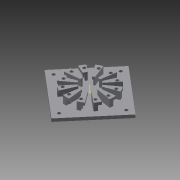
# Autodesk Inventor part: male bayonet connector 12
Saved by Autodesk Inventor 2015 (Build 190159000, 159)
## iProperties
Created: 2014-06-11
Part Number: male bayonet connector 12
Material: Generic
Document SubType Name: Modeling
Designer: ericd_000
Density: 1 g/cm^3
Appearance: Default
Author: ericd_000
Autodesk Inventor part; units mm, degrees
ref_plane "YZ Plane" through (0, 0, 0) normal (1, 0, 0) x (0, 1, 0)
ref_plane "XZ Plane" through (0, 0, 0) normal (0, 1, 0) x (-1, 0, 0)
ref_plane "XY Plane" through (0, 0, 0) normal (0, 0, 1) x (1, 0, 0)
sketch "Sketch19" plane through (0, 0, 0) normal (0, 0, 1) x (1, 0, 0)
  circle A0 centre (0, 0) radius 39.5
  dimension "d94" = 79
  constraints: 1 centre point, 1 coincident
  measures "d94" diameter of A0
extrude "Extrusion20" add sketch "Sketch19" along normal blind 5
sketch "Sketch21" plane through (0, 0, 5) normal (0, 0, 1) x (1, 0, 0)
  point P0 (0, 0)
sketch "Sketch23" plane through (0, 0, 5) normal (0, 0, 1) x (1, 0, 0)
  line L0 (0, 0) -> (20.2843, 33.8939) construction
  circle A0 centre (0, 0) radius 39.5 construction
  line L1 (0, 0) -> (24.804, 30.7411) construction
  circle A1 centre (0, 0) radius 39.5 construction
  line L2 (24.804, 30.7411) -> (9.4735, 11.7411)
  line L3 (9.4735, 11.7411) -> (7.6719, 12.8193)
  line L4 (7.6719, 12.8193) -> (20.2843, 33.8939)
  arc A2 (24.804, 30.7411) -> (20.2843, 33.8939) centre (0, 0) ccw
  dimension "d105" = 172
  dimension "d106" = 19
  constraints: 10 end point, 2 collinear, 2 point on circle, 1 centre point, 1 perpendicular, 5 other
  measures "d105" angle of L0 L1
  measures "d106" vertical distance of L1.end L2.end
extrude "Extrusion21" add sketch "Sketch23" along normal blind 12.5
sketch "Sketch26" plane through (7.6719, 12.8193, 5) normal (-0.8580744, 0.5135254, 0) x (0, 0, 1)
  line L0 (12.5, 24.5604) -> (12.5, 0)
  line L1 (12.5, 24.5604) -> (8.1, 24.5604)
  line L2 (0, 24.5604) -> (12.5, 24.5604) projected
  line L3 (0, 0) -> (12.5, 0) projected
  line L4 (8.1, 0) -> (12.5, 0)
  line L5 (8.1, 24.5604) -> (8.1, 0)
  line L6 (-8.5, -14.9396) -> (16, -14.9396) projected
  line L7 (12.5, 24.5604) -> (12.5, 0) projected
  point P0 (-5, -14.9396)
  dimension "d123" = 4.4
  constraints: 8 end point, 2 point on line, 1 collinear, 1 parallel, 1 vertical
  measures "d123" distance of L4.start L0.end
revolve "Revolution2" add sketch "Sketch26" angle 7 about axis through (0, 0, 5) along (0, 0, 1)
sketch "Sketch25" plane through (0, 0, 17.5) normal (0, 0, 1) x (1, 0, 0)
  circle A0 centre (18.2106, 27.5205) radius 2.5
  line L0 (18.2106, 27.5205) -> (0, 0) construction
  line L1 (6.0524, 13.6587) -> (16.0024, 36.1133) projected
  dimension "d112" = 5
  dimension "d116" = 33
  dimension "d125" = 5.5
  constraints: 2 end point, 1 centre point
  measures "d112" diameter of A0
  measures "d116" distance of L0.start L0.end
  measures "d125" distance from line of L0.start L1
extrude "Extrusion22" cut sketch "Sketch25" against normal through all
sketch "Sketch27" plane through (0, 0, 17.5) normal (0, 0, 1) x (1, 0, 0)
  line L0 (7.6719, 12.8193) -> (9.4735, 11.7411) projected
  line L1 (7.6719, 12.8193) -> (6.0524, 13.6587)
  line L2 (6.0524, 13.6587) -> (20.1635, 45.5037)
  line L3 (6.0524, 13.6587) -> (16.0024, 36.1133) projected
  line L4 (20.1635, 45.5037) -> (7.6753, 12.8175)
  point P0 (0, 0)
  constraints: 7 end point, 2 point on line
extrude "Extrusion23" [suppressed]
pattern_circular "Circular Pattern2" count 12 over 360 about axis through (0, 0, 5) along (0, 0, 1) of "Extrusion21", "Revolution2", "Extrusion22"
sketch "Sketch29" plane through (0, 0, 5) normal (0, 0, 1) x (1, 0, 0)
  circle A0 centre (0, 0) radius 59
  line L0 (0, 0) -> (-30.7411, 24.804)
  line L1 (0, 0) -> (-33.8939, 20.2843)
  line L2 (-12.8193, 7.6719) -> (-33.8939, 20.2843) projected
  arc A1 (-34.5136, -19.2109) -> (-24.804, -30.7411) centre (0, 0) ccw projected
  point P0 (-30.0077, 17.9585)
  dimension "d135" = 118
  constraints: 4 end point, 1 centre point, 1 coincident, 1 collinear, 1 concentric
  measures "d135" diameter of A0
extrude "Extrusion26" [suppressed]
sketch "Sketch30" plane through (0, 0, 5) normal (0, 0, -1) x (-1, 0, 0)
  line L0 (-109.7485, 105.489) -> (97.8298, 105.489)
  line L1 (97.8298, 105.489) -> (97.8298, -69.3705)
  line L2 (97.8298, -69.3705) -> (-109.7485, -69.3705)
  line L3 (-109.7485, -69.3705) -> (-109.7485, 105.489)
  line L4 (10.1144, -4.0386) -> (9.0138, 1.6159)
  line L5 (9.0138, 1.6159) -> (50.6067, 20.2684)
  line L6 (50.6067, 20.2684) -> (50.6067, -5.7642)
  line L7 (50.6067, -5.7642) -> (10.1144, -4.0386)
  point P0 (0, 0)
  constraints: 16 end point, 2 parallel, 1 horizontal, 1 perpendicular, 1 vertical
extrude "Extrusion27" [suppressed]
sketch "Sketch31" plane through (-36.1133, 16.0024, 17.5) normal (0, 0, 1) x (0.9142614, -0.4051247, 0)
  line L0 (16, 0) -> (20, 0)
  line L1 (20, 0) -> (20, 3)
  line L2 (20, 3) -> (16, 3)
  line L3 (16, 3) -> (16, 0)
  line L4 (24.5604, 0) -> (0, 0) projected
  point P0 (39.5, 0)
  point P1 (24.7502, 0)
  dimension "d148" = 16
  dimension "d149" = 4
  dimension "d150" = 3
  constraints: 8 end point, 2 parallel, 1 collinear, 1 horizontal, 1 perpendicular
  measures "d148" distance from line of L3 L4.end
  measures "d149" distance of L1.end L2.end
  measures "d150" distance of L0.end L1.end
extrude "Extrusion28" cut sketch "Sketch31" against normal up to surface (4.4 mm away)
sketch "Sketch32" plane through (-30.7411, 24.804, 17.5) normal (0, 0, 1) x (0.7782548, -0.6279487, 0)
  line L0 (16.8007, -6.0822) -> (15.171, 0)
  line L1 (0, 0) -> (24.4136, 0) projected
  line L2 (16.8007, -6.0822) -> (16.0243, -3.1845) projected
  line L3 (16.8007, -6.0822) -> (25.0695, -3.8666)
  line L4 (25.0695, -3.8666) -> (24.4136, 0)
  line L5 (15.171, 0) -> (24.4136, 0)
  line L6 (16.8007, -6.0822) -> (16.511, -6.1599)
  line L7 (16.8007, -6.0822) -> (1.3459, -10.2234) projected
  line L8 (14.8604, 0) -> (15.171, 0)
  line L9 (15.171, 0) -> (14.8604, 0)
  line L10 (16.511, -6.1599) -> (14.8604, 0)
  point P0 (39.5, 0)
  point P1 (8.718, -8.248)
  dimension "d153" = 0.3
  constraints: 16 end point, 4 collinear, 3 point on line, 1 parallel
  measures "d153" distance between parallel lines of L10 L0
extrude "Extrusion30" cut sketch "Sketch32" against normal up to surface (12.5 mm away)
sketch "Sketch33" plane through (0, 0, 0) normal (0, 0, -1) x (-1, 0, 0)
  circle A0 centre (0, 0) radius 39.5
  line L0 (5.7901, 70.4732) -> (-70.4732, 5.7901)
  line L1 (-70.4732, 5.7901) -> (-5.7901, -70.4732)
  line L2 (-5.7901, -70.4732) -> (70.4732, -5.7901)
  line L3 (70.4732, -5.7901) -> (5.7901, 70.4732)
  line L4 (-38.1317, -32.3415) -> (38.1317, 32.3415) construction
  line L5 (32.3415, -38.1317) -> (-32.3415, 38.1317) construction
  point P0 (0, -32.0404)
  point P1 (67.1306, 0)
  point P2 (-36.4741, 21.0583)
  point P3 (30.6565, 53.0987)
  dimension "d171" = 79
  dimension "d191" = 100
  dimension "d192" = 100
  constraints: 12 end point, 6 midpoint, 2 parallel, 1 centre point, 1 coincident, 1 horizontal alignment, 1 perpendicular, 1 vertical alignment
  measures "d171" diameter of A0
  measures "d191" distance of L1.end L2.end
  measures "d192" distance of L2.end L0.start
sketch "Sketch34" plane through (0, 0, 5) normal (0, 0, 1) x (1, 0, 0)
  point P0 (0, 0)
extrude "Extrusion34" add sketch "Sketch33" against normal blind 5
sketch "Sketch35" plane through (0, 0, 0) normal (0, 0, -1) x (-1, 0, 0)
  line L0 (-70.4732, 5.7901) -> (5.7901, 70.4732)
  line L1 (5.7901, 70.4732) -> (70.4732, -5.7901) projected
  line L2 (5.7901, 70.4732) -> (70.4732, -5.7901)
  line L3 (70.4732, -5.7901) -> (-5.7901, -70.4732)
  line L4 (-5.7901, -70.4732) -> (-70.4732, 5.7901)
  line L5 (-5.7901, -70.4732) -> (-70.4732, 5.7901) projected
  circle A0 centre (-56.3786, 4.6321) radius 2.5
  circle A1 centre (4.6321, 56.3786) radius 2.5
  circle A2 centre (-4.6321, -56.3786) radius 2.5
  circle A3 centre (56.3786, -4.6321) radius 2.5
  point P0 (0, 0)
  dimension "d188" = 10
  dimension "d189" = 10
  dimension "d190" = 5
  dimension "d195" = 80
  dimension "d198" = 80
  constraints: 8 end point, 4 centre point, 2 collinear, 2 perpendicular, 8 other
  measures "d188" distance from line of L0 A0.centre
  measures "d189" distance from line of L4 A0.centre
  measures "d190" diameter of A0
  measures "d195" distance of A0.centre A1.centre
  measures "d198" distance of A0.centre A2.centre
extrude "Extrusion35" cut sketch "Sketch35" against normal blind 5 contours A0 | A1 | A2 | A3
body "Solid2"
